Diaper Place Single (Autodesk Fusion 360 design; units mm, degrees)
Autodesk Fusion 360 part; units mm, degrees
note: some values were not read from the file. Set by a fixed rule: which sketch regions a step uses.
sketch "Sketch1" plane through (0, 0, 0) normal (0, 0, 1) x (1, 0, 0)
  line L0 (0, 0) -> (1615, 0)
  line L1 (1615, 0) -> (1615, 505)
  line L2 (1615, 505) -> (0, 505)
  line L3 (0, 505) -> (0, 0)
  line L4 (50, 493) -> (1565, 493)
  line L5 (1565, 493) -> (1565, 15)
  line L6 (1565, 15) -> (50, 15)
  line L7 (50, 15) -> (50, 493)
  dimension "d1" = 505
  dimension "d2" = 1615
  dimension "d3" = 12
  dimension "d4" = 50
  dimension "d5" = 50
  dimension "d6" = 15
  constraint horizontal L0
  constraint vertical L1
  constraint horizontal L2
  constraint vertical L3
  constraint coincident L0.start L3.end
  constraint horizontal L4
  constraint vertical L5
  constraint horizontal L6
  constraint vertical L7
  measures "d1" distance of L0.start L2.end
  measures "d2" distance of L1.end L2.end
  measures "d3" distance of L2 L4
  measures "d4" distance of L3 L7
  measures "d5" distance of L1 L5
  measures "d6" distance of L0 L6
extrude "Extrude1" add sketch "Sketch1" along normal blind 23 contours L0 L1 L2 L3 | L4 L5 L6 L7 makes body 1
extrude "Extrude2" add sketch "Sketch1" against normal blind 942 contours L4 L5 L6 L7 bodies 1
sketch "Sketch2" plane through (0, 0, 23) normal (0, 0, 1) x (-1, 0, 0)
  line L0 (0, -505) -> (0, 0)
  line L1 (0, 0) -> (-1615, 0)
  line L2 (-1615, 0) -> (-1615, -505)
  line L3 (-1615, -505) -> (0, -505)
  line L4 (-517.9302, -505) -> (-1267.9302, -505)
  line L5 (-1267.9302, -505) -> (-1267.9302, 195)
  line L6 (-1267.9302, 195) -> (-517.9302, 195)
  line L7 (-517.9302, 195) -> (-517.9302, -505)
  line L8 (-1615, -505) -> (0, -505)
  dimension "d11" = 750
  dimension "d12" = 700
  constraint horizontal L4
  constraint vertical L5
  constraint horizontal L6
  constraint vertical L7
  constraint coincident L4.start L8
  measures "d11" distance of L4.start L4.end
  measures "d12" distance of L4.start L6.end
extrude "Extrude3" add sketch "Sketch2" along normal blind 15 separate body contours L1 L3 L4 L5 L7 L8 | L1 L5 L6 L7 makes body 2
sketch "Sketch3" plane through (1267.9302, 0, 0) normal (1, 0, 0) x (0, 1, 0)
  line L0 (-195, 23) -> (505, 23)
  line L1 (505, 23) -> (505, 38)
  line L2 (505, 38) -> (-195, 38)
  line L3 (505, 23) -> (-195, 23)
  line L4 (-195, 23) -> (-195, 138)
  line L5 (-195, 138) -> (505, 138)
  line L6 (505, 138) -> (505, 23)
  line L7 (-195, 38) -> (-195, 23)
  dimension "d21" = 700
  dimension "d22" = 115
  constraint horizontal L3
  constraint vertical L4
  constraint horizontal L5
  constraint vertical L6
  constraint coincident L0.end L1.start
  measures "d21" distance of L0.end L0.start
  measures "d22" distance of L0.end L5.end
extrude "Extrude5" add sketch "Sketch3" along normal blind 15 separate body makes body 3
extrude "Extrude6" add sketch "Sketch3" along normal blind 15 from surface at -765 separate body makes body 4
sketch "Sketch6" plane through (0, 505, 0) normal (0, 1, 0) x (-1, 0, 0)
  line L0 (-1615, 0) -> (0, 0)
  line L1 (0, 0) -> (0, 23)
  line L2 (0, 23) -> (-1615, 23)
  line L3 (-1615, 23) -> (-1615, 0)
  line L4 (-1282.9302, 138) -> (-502.9302, 138)
  line L5 (-502.9302, 138) -> (-502.9302, -15)
  line L6 (-502.9302, -15) -> (-1282.9302, -15)
  line L7 (-1282.9302, -15) -> (-1282.9302, 138)
  point P0 (-1282.9302, 138)
  point P1 (-502.9302, 138)
  dimension "d29" = 15
  constraint horizontal L4
  constraint vertical L5
  constraint horizontal L6
  constraint vertical L7
  constraint coincident P0 L4.start
  constraint coincident P1 L4.end
  measures "d29" distance of L0 L6
extrude "Extrude7" add sketch "Sketch6" along normal blind 15 separate body contours L0 L2 L5 L7 | L0 L5 L6 L7 | L2 L4 L5 L7 makes body 5
fillet "Fillet1" radius 85 2 edges at (1275.4302, -195, 138) (510.4302, -195, 138) on bodies 3 4
equation "d11 = base_width"
equation "d12 = base_height"
equation "base_width = 750 mm"
equation "base_height = 700 mm"
equation "material_thickness = 15 mm"
equation "d17 = material_thickness"
equation "d21 = base_height"
equation "d22 = base_sidewalls + material_thickness"
equation "base_sidewalls = 100 mm"
equation "d24 = material_thickness"
equation "d26 = -( base_width + material_thickness )"
equation "d27 = material_thickness"
equation "d29 = material_thickness"
equation "d30 = material_thickness"
equation "d33 = base_sidewalls - material_thickness"
named bodies: "Schrank", "base back", "base side right", "base side left", "base side back"
